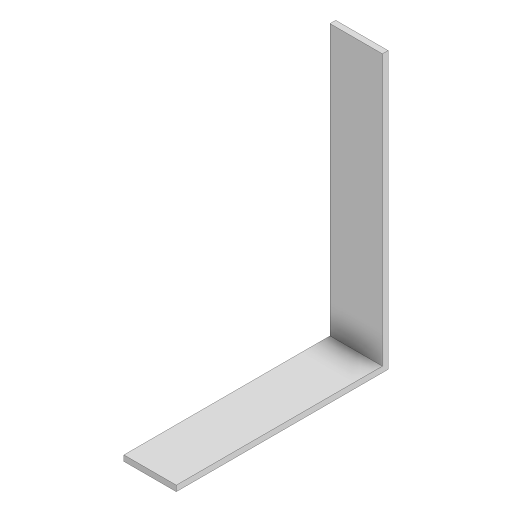
# Autodesk Inventor part: PLETINA NEMA CAJA
Saved by Autodesk Inventor 2024 (Build 280153000, 153)
## iProperties
Created: 2024-07-05
Part Number: PLETINA NEMA CAJA
Material: Generic
Document SubType Name: Modeling
Designer: Jhuliams
Density: 1 g/cm^3
Appearance: Default
Author: Jhuliams
Autodesk Inventor part; units mm, degrees
ref_plane "YZ Plane" through (0, 0, 0) normal (1, 0, 0) x (0, 1, 0)
ref_plane "XZ Plane" through (0, 0, 0) normal (0, 1, 0) x (-1, 0, 0)
ref_plane "XY Plane" through (0, 0, 0) normal (0, 0, 1) x (1, 0, 0)
sketch "Sketch1" plane through (0, 0, 0) normal (1, 0, 0) x (0, 1, 0)
  line L0 (0, 0) -> (134, 0)
  line L1 (134, 0) -> (134, -2.75)
  line L2 (134, -2.75) -> (0, -2.75)
  line L3 (0, -2.75) -> (0, 0)
  line L4 (0, 0) -> (2.75, 0)
  line L5 (2.75, 0) -> (2.75, 100)
  line L6 (2.75, 100) -> (0, 100)
  line L7 (0, 100) -> (0, 0)
  dimension "d0" = 134
  dimension "d1" = 2.75
  dimension "d2" = 2.75
  dimension "d3" = 100
  constraints: 16 end point, 4 parallel, 2 horizontal, 2 perpendicular
  measures "d0" distance of L1.end L2.end
  measures "d1" distance of L0.end L1.end
  measures "d2" distance of L6.end L5.end
  measures "d3" distance of L5.end L4.end
extrude "Extrusion1" add sketch "Sketch1" against normal blind 25.4
body "Solid1"
